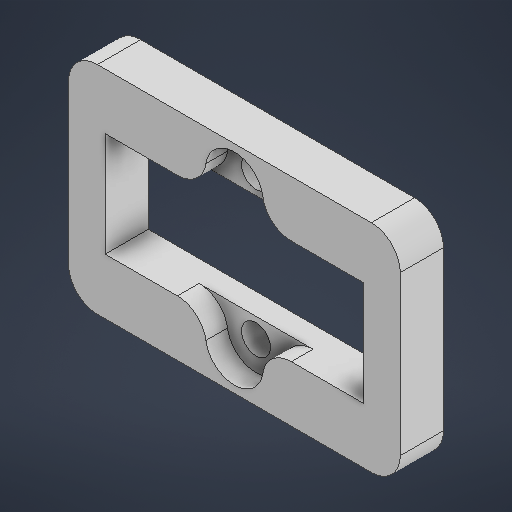
# Autodesk Inventor part: 4mm隔热板
Saved by Autodesk Inventor 2025 (Build 290162000, 162)
## iProperties
Created: 2025-03-08
Part Number: 4mm隔热板
Material: 常规
Document SubType Name: Modeling
Designer: XH
Density: 1 g/cm^3
Appearance: 默认
Author: XH
Autodesk Inventor part; units mm, degrees
ref_plane "YZ Plane" through (0, 0, 0) normal (1, 0, 0) x (0, 1, 0)
ref_plane "XZ Plane" through (0, 0, 0) normal (0, 1, 0) x (-1, 0, 0)
ref_plane "XY Plane" through (0, 0, 0) normal (0, 0, 1) x (1, 0, 0)
sketch "草图1" plane through (0, 0, 0) normal (0, 0, 1) x (1, 0, 0)
  line L0 (11.5, -7.5) -> (-11.5, -7.5)
  line L1 (-11.5, -7.5) -> (-11.5, 7.5)
  line L2 (-11.5, 7.5) -> (11.5, 7.5)
  line L3 (11.5, 7.5) -> (11.5, -7.5)
  line L4 (11.5, -7.5) -> (-11.5, 7.5) construction
  line L5 (-11.5, -7.5) -> (11.5, 7.5) construction
  point P0 (0, 0)
  dimension "d0" = 23
  dimension "d1" = 15
  constraints: 12 end point, 2 midpoint, 2 parallel, 1 horizontal, 1 perpendicular
  measures "d0" distance of L1.end L2.end
  measures "d1" distance of L0.end L1.end
extrude "拉伸1" add sketch "草图1" along normal blind 3
sketch "草图2" plane through (0, 0, 3) normal (0, 0, 1) x (1, 0, 0)
  circle A0 centre (0, 5) radius 1
  point P0 (0, 0)
  dimension "d4" = 2
  dimension "d10" = 5
  constraints: 1 centre point
  measures "d4" diameter of A0
  measures "d10" distance of A0.centre point (0, 0)
extrude "拉伸2" cut sketch "草图2" against normal blind 4
sketch "草图3" plane through (0, 0, 0) normal (0, 0, -1) x (-1, 0, 0)
  line L0 (8.9655, -3.6241) -> (-8.9655, -3.6241)
  line L1 (-8.9655, -3.6241) -> (-8.9655, 3.6241)
  line L2 (-8.9655, 3.6241) -> (8.9655, 3.6241)
  line L3 (8.9655, 3.6241) -> (8.9655, -3.6241)
  line L4 (8.9655, -3.6241) -> (-8.9655, 3.6241) construction
  line L5 (-8.9655, -3.6241) -> (8.9655, 3.6241) construction
  point P0 (0, 0)
  constraints: 12 end point, 2 midpoint, 2 parallel, 1 horizontal, 1 perpendicular
extrude "拉伸3" cut sketch "草图3" against normal blind 4
fillet "圆角1" radius 2 4 edges at (11.5, 7.5, 1.5) (-11.5, 7.5, 1.5) (-11.5, -7.5, 1.5) (11.5, -7.5, 1.5)
sketch "草图4" plane through (0, 0, 3) normal (0, 0, 1) x (1, 0, 0)
  circle A0 centre (0, 5) radius 1 projected
  circle A1 centre (0, 5) radius 2
  point P0 (0, 0)
  dimension "d11" = 4
  constraints: 1 centre point, 1 coincident
  measures "d11" diameter of A1
extrude "拉伸4" cut sketch "草图4" against normal blind 1.5 contours A0 | A1
fillet "圆角2" radius 2 2 edges at (1.4515, 3.6241, 2.25) (-1.4515, 3.6241, 2.25)
mirror "镜像1" about plane through (0, 0, 0) normal (0, 1, 0) of "拉伸4", "圆角2", "拉伸2"
